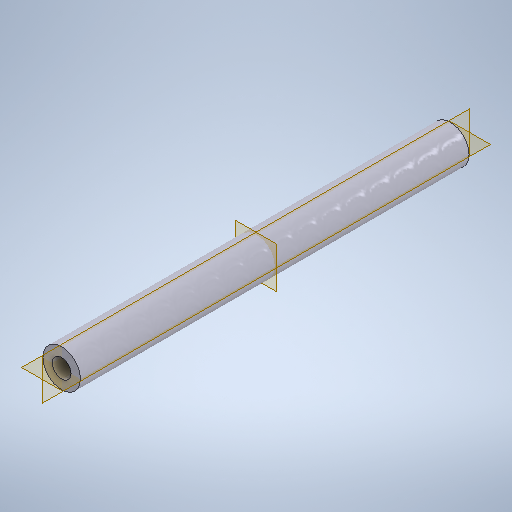
# Autodesk Inventor part: Sessao7_02_04_2025_0002_001
Saved by Autodesk Inventor 2025.2 (Build 292293000, 293)
## iProperties
Created: 2025-04-02
Part Number: Sessao7_02_04_2025_0002_001
Material: Aço inoxidável
Document SubType Name: Modeling
Designer: lucas
Density: 8 g/cm^3
Appearance: Aço inoxidável - Soldado
Author: lucas
Autodesk Inventor part; units mm, degrees
sketch "Esboço1" plane through (0, 0, 0) normal (0, 0, 1) x (1, 0, 0)
  circle A0 centre (0, 0) radius 35
  circle A1 centre (0, 0) radius 17.5
  dimension "d0" = 70
  dimension "d1" = 35
  constraints: 2 centre point, 2 coincident
  measures "d0" diameter of A0
  measures "d1" diameter of A1
extrude "Extrusão1" add sketch "Esboço1" along normal mid plane 725
